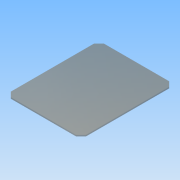
# Autodesk Inventor part: крышка 2
Saved by Autodesk Inventor 2017 (Build 210142000, 142)
## iProperties
Part Number: крышка 2
Material: Типовые
Document SubType Name: Modeling
Designer: Max
Mass: 260.283 g
Surface Area: 1343.49 cm^2
Volume: 260.283 cm^3
Density: 1 g/cm^3
Appearance: Поликарбонат — дымчатый
Author: Max
Autodesk Inventor part; units mm, degrees
ref_plane "YZ Plane" through (0, 0, 0) normal (1, 0, 0) x (0, 1, 0)
ref_plane "XZ Plane" through (0, 0, 0) normal (0, 1, 0) x (-1, 0, 0)
ref_plane "XY Plane" through (0, 0, 0) normal (0, 0, 1) x (1, 0, 0)
sketch "Эскиз1" plane through (0, 0, 0) normal (0, 0, 1) x (1, 0, 0)
  line L0 (-168.7947, 191.7053) -> (-168.7947, -196.2947) projected
  line L1 (-168.7947, -196.2947) -> (170.2053, -196.2947) projected
  line L2 (170.2053, -196.2947) -> (170.2053, 191.7053) projected
  line L3 (170.2053, 191.7053) -> (-168.7947, 191.7053) projected
  line L4 (-120.597, 140.6454) -> (109.403, 140.6454)
  line L5 (109.403, 140.6454) -> (109.403, -144.3546)
  line L6 (109.403, -144.3546) -> (-120.597, -144.3546)
  line L7 (-120.597, -144.3546) -> (-120.597, 140.6454)
  line L8 (109.903, 141.1454) -> (109.903, -144.8546) projected
  line L9 (109.903, -144.8546) -> (-121.097, -144.8546) projected
  line L10 (-121.097, -144.8546) -> (-121.097, 141.1454) projected
  line L11 (-121.097, 141.1454) -> (109.903, 141.1454) projected
  line L12 (170.903, -196.8546) -> (170.903, 193.1454) projected
  line L13 (170.903, 193.1454) -> (-173.097, 193.1454) projected
  line L14 (-173.097, 193.1454) -> (-173.097, -196.8546) projected
  line L15 (-173.097, -196.8546) -> (170.903, -196.8546) projected
  point P0 (0, 0)
  dimension "d6" = 0.5
  dimension "d7" = 0.5
  dimension "d8" = 0.5
  dimension "d9" = 0.5
  constraints: 8 end point, 2 parallel, 1 horizontal, 1 perpendicular
  measures "d6" distance between parallel lines of L11 L4
  measures "d7" distance between parallel lines of L5 L8
  measures "d8" distance between parallel lines of L9 L6
  measures "d9" distance between parallel lines of L10 L7
extrude "Выдавливание1" add sketch "Эскиз1" against normal blind 4 contours L4 L5 L6 L7
chamfer "Фаска1" distance 14.78 angle 45 4 edges at (-120.597, -144.3546, -2) (109.403, -144.3546, -2) (109.403, 140.6454, -2) (-120.597, 140.6454, -2)
sketch "Эскиз2" plane through (0, 0, -4) normal (0, 0, -1) x (-1, 0, 0)
  circle A0 centre (-95.653, -94.8546) radius 1.5 projected
  circle A1 centre (-95.653, -64.8546) radius 1.5 projected
  circle A2 centre (-95.653, 61.1454) radius 1.5 projected
  circle A3 centre (-95.653, 91.1454) radius 1.5 projected
  line L0 (-109.403, 125.8654) -> (-109.403, -129.5746) projected
  point P0 (0, 0)
  dimension "d13" = 3
  dimension "d16" = 30
  dimension "d17" = 13.75
  measures "d13" diameter of A2
  measures "d16" distance of A1.centre A0.centre
  measures "d17" distance from line of L0 A0.centre
extrude "Выдавливание2" cut sketch "Эскиз2" against normal blind 10
sketch "Эскиз3" plane through (0, 0, 0) normal (0, 0, 1) x (1, 0, 0)
  line L0 (0, 0) -> (-163.3062, 0) construction
  circle A0 centre (-105.597, -10) radius 1.5
  circle A1 centre (-105.597, 10) radius 1.5
  line L1 (-120.597, -129.5746) -> (-120.597, 125.8654) projected
  dimension "d18" = 3
  dimension "d19" = 3
  dimension "d20" = 20
  dimension "d21" = 15
  constraints: 2 centre point, 2 end point, 1 horizontal, 1 symmetric about line
  measures "d18" diameter of A0
  measures "d19" diameter of A1
  measures "d20" distance of A0.centre A1.centre
  measures "d21" distance from line of L1 A0.centre
extrude "Выдавливание3" cut sketch "Эскиз3" against normal blind 10
